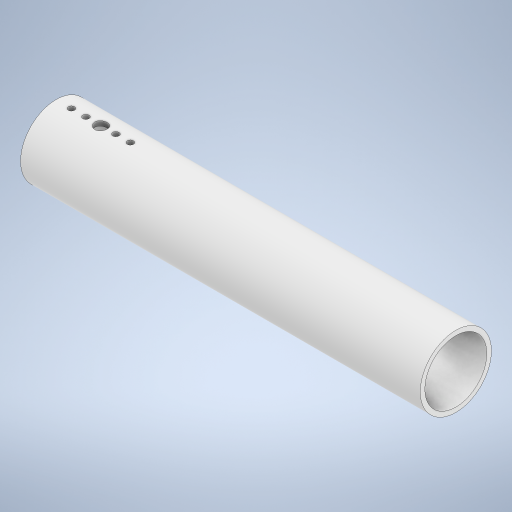
# Autodesk Inventor part: Arm Segment 2
Saved by Autodesk Inventor 2023 (Build 270158030, 158C)
## iProperties
Created: 2022-10-01
Part Number: Arm Segment 2
Material: PVC-Piping
Document SubType Name: Modeling
Designer: cjj5381
Density: 1.4 g/cm^3
Appearance: Smooth - White
Author: cjj5381
Autodesk Inventor part; units mm, degrees
ref_plane "YZ Plane" through (0, 0, 0) normal (1, 0, 0) x (0, 1, 0)
ref_plane "XZ Plane" through (0, 0, 0) normal (0, 1, 0) x (-1, 0, 0)
ref_plane "XY Plane" through (0, 0, 0) normal (0, 0, 1) x (1, 0, 0)
sketch "Sketch1" plane through (0, 0, 0) normal (1, 0, 0) x (0, 1, 0)
  circle A0 centre (0, 0) radius 26.2509
  circle A1 centre (0, 0) radius 30.1625
  dimension "d0" = 52.5018
  dimension "d1" = 3.9116
  constraints: 2 centre point, 1 coincident
  measures "d0" diameter of A0
  measures "d1" radial gap between concentric circles of A0 A1
extrude "Extrusion1" add sketch "Sketch1" along normal mid plane 339
sketch "Sketch2" plane through (0, 0, 0) normal (0, 1, 0) x (1, 0, 0)
  circle A0 centre (-131.4, 0) radius 5.25
  line L0 (-169.5, -26.2509) -> (-169.5, 26.2509) projected
  point P0 (0, 0)
  dimension "d4" = 10.5
  dimension "d5" = 38.1
  constraints: 1 centre point
  measures "d4" diameter of A0
  measures "d5" distance from line of L0 A0.centre
extrude "Extrusion2" cut sketch "Sketch2" along normal through all both and the other way through all
sketch "Sketch3" plane through (0, 0, 0) normal (0, 1, 0) x (-1, 0, 0)
  circle A0 centre (156.5, 0) radius 2.625
  circle A1 centre (106.5, 0) radius 2.6358
  line L0 (0, 0) -> (162.823, 0) construction
  line L1 (131.5, 0) -> (131.5, -16.0563) construction
  line L2 (169.5, 26.2509) -> (169.5, -26.2509) construction
  circle A2 centre (144.2, 0) radius 2.625
  circle A3 centre (118.8, 0) radius 2.625
  dimension "d8" = 5.25
  dimension "d9" = 50
  dimension "d10" = 38
  dimension "d13" = 5.25
  dimension "d14" = 25.4
  constraints: 5 point on line, 4 centre point, 4 end point, 2 symmetric about line, 1 equal radius, 1 horizontal, 1 vertical
  measures "d8" diameter of A0
  measures "d9" distance of A1.centre A0.centre
  measures "d10" distance between parallel lines of L2 L1
  measures "d13" diameter of A3
  measures "d14" distance of A2.centre A3.centre
extrude "Extrusion3" cut sketch "Sketch3" along normal through all both and the other way through all
body "Solid1"
